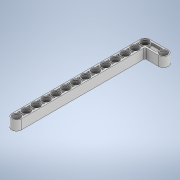
# Autodesk Inventor part: gear-rack
Saved by Autodesk Inventor 2021 (Build 250183000, 183)
## iProperties
Created: 2024-04-11
Part Number: gear-rack
Material: Generic
Document SubType Name: Modeling
Designer: 22hamfri
Density: 1 g/cm^3
Appearance: Default
Author: 22hamfri
Autodesk Inventor part; units mm, degrees
ref_plane "YZ Plane" through (0, 0, 0) normal (1, 0, 0) x (0, 1, 0)
ref_plane "XZ Plane" through (0, 0, 0) normal (0, 1, 0) x (-1, 0, 0)
ref_plane "XY Plane" through (0, 0, 0) normal (0, 0, 1) x (1, 0, 0)
sketch "Sketch1" plane through (0, 0, 0) normal (0, 1, 0) x (-1, 0, 0)
  circle A0 centre (0, 0) radius 2.575
  circle A1 centre (0, 0) radius 3.1
  circle A2 centre (0, 0) radius 3.8
  circle A3 centre (-14.94, 0) radius 2.575
  circle A4 centre (-14.94, 0) radius 3.1
  circle A5 centre (-14.94, 0) radius 3.8
  line L0 (0, -3.8) -> (-14.94, -3.8)
  line L1 (-4.8, 3.8) -> (-14.94, 3.8)
  line L2 (0, 0) -> (-14.94, 0)
  line L3 (0, 0) -> (0, 103.61)
  circle A6 centre (0, 7.97) radius 2.575
  circle A7 centre (0, 7.97) radius 3.1
  circle A8 centre (0, 7.97) radius 3.8
  circle A9 centre (0, 15.94) radius 2.575
  circle A10 centre (0, 15.94) radius 3.1
  circle A11 centre (0, 15.94) radius 3.8
  circle A12 centre (0, 23.91) radius 2.575
  circle A13 centre (0, 23.91) radius 3.1
  circle A14 centre (0, 23.91) radius 3.8
  circle A15 centre (0, 31.88) radius 2.575
  circle A16 centre (0, 31.88) radius 3.1
  circle A17 centre (0, 31.88) radius 3.8
  circle A18 centre (0, 39.85) radius 2.575
  circle A19 centre (0, 39.85) radius 3.1
  circle A20 centre (0, 39.85) radius 3.8
  circle A21 centre (0, 47.82) radius 2.575
  circle A22 centre (0, 47.82) radius 3.1
  circle A23 centre (0, 47.82) radius 3.8
  circle A24 centre (0, 55.79) radius 2.575
  circle A25 centre (0, 55.79) radius 3.1
  circle A26 centre (0, 55.79) radius 3.8
  circle A27 centre (0, 63.76) radius 2.575
  circle A28 centre (0, 63.76) radius 3.1
  circle A29 centre (0, 63.76) radius 3.8
  circle A30 centre (0, 71.73) radius 2.575
  circle A31 centre (0, 71.73) radius 3.1
  circle A32 centre (0, 71.73) radius 3.8
  circle A33 centre (0, 79.7) radius 2.575
  circle A34 centre (0, 79.7) radius 3.1
  circle A35 centre (0, 79.7) radius 3.8
  circle A36 centre (0, 87.67) radius 2.575
  circle A37 centre (0, 87.67) radius 3.1
  circle A38 centre (0, 87.67) radius 3.8
  circle A39 centre (0, 95.64) radius 2.575
  circle A40 centre (0, 95.64) radius 3.1
  circle A41 centre (0, 95.64) radius 3.8
  circle A42 centre (0, 103.61) radius 2.575
  circle A43 centre (0, 103.61) radius 3.1
  circle A44 centre (0, 103.61) radius 3.8
  line L4 (3.8, 103.61) -> (3.8, 0)
  line L5 (-3.8, 4.8) -> (-3.8, 103.61)
  line L6 (-3.0249, -2.3) -> (-11.9151, -2.3)
  line L7 (-3.0249, 2.3) -> (-11.9151, 2.3)
  line L8 (-2.3, 100.5851) -> (-2.3, 98.6649)
  line L9 (-2.3, 92.6151) -> (-2.3, 90.6949)
  line L10 (-2.3, 84.6451) -> (-2.3, 82.7249)
  line L11 (-2.3, 76.6751) -> (-2.3, 74.7549)
  line L12 (-2.3, 68.7051) -> (-2.3, 66.7849)
  line L13 (-2.3, 60.7351) -> (-2.3, 58.8149)
  line L14 (-2.3, 52.7651) -> (-2.3, 50.8449)
  line L15 (-2.3, 44.7951) -> (-2.3, 42.8749)
  line L16 (-2.3, 36.8251) -> (-2.3, 34.9049)
  line L17 (-2.3, 28.8551) -> (-2.3, 26.9349)
  line L18 (-2.3, 20.8851) -> (-2.3, 18.9649)
  line L19 (-2.3, 12.9151) -> (-2.3, 10.9949)
  line L20 (-2.3, 4.9451) -> (-2.3, 3.0249)
  line L21 (2.3, 100.5851) -> (2.3, 98.6649)
  line L22 (2.3, 92.6151) -> (2.3, 90.6949)
  line L23 (2.3, 84.6451) -> (2.3, 82.7249)
  line L24 (2.3, 76.6751) -> (2.3, 74.7549)
  line L25 (2.3, 68.7051) -> (2.3, 66.7849)
  line L26 (2.3, 60.7351) -> (2.3, 58.8149)
  line L27 (2.3, 52.7651) -> (2.3, 50.8449)
  line L28 (2.3, 44.7951) -> (2.3, 42.8749)
  line L29 (2.3, 36.8251) -> (2.3, 34.9049)
  line L30 (2.3, 28.8551) -> (2.3, 26.9349)
  line L31 (2.3, 20.8851) -> (2.3, 18.9649)
  line L32 (2.3, 12.9151) -> (2.3, 10.9949)
  line L33 (2.3, 4.9451) -> (2.3, 3.0249)
  arc A45 (-4.8, 3.8) -> (-3.8, 4.8) centre (-4.8, 4.8) ccw
  point P0 (0, 3.8)
  point P1 (0, 4.17)
  point P2 (0, 11.77)
  point P3 (0, 12.14)
  point P4 (0, 19.74)
  point P5 (0, 20.11)
  point P6 (0, 27.71)
  point P7 (0, 28.08)
  point P8 (0, 35.68)
  point P9 (0, 36.05)
  point P10 (0, 43.65)
  point P11 (0, 44.02)
  point P12 (0, 51.62)
  point P13 (0, 51.99)
  point P14 (0, 59.59)
  point P15 (0, 59.96)
  point P16 (0, 67.56)
  point P17 (0, 67.93)
  point P18 (0, 75.53)
  point P19 (0, 75.9)
  point P20 (0, 83.5)
  point P21 (0, 83.87)
  point P22 (0, 91.47)
  point P23 (0, 91.84)
  point P24 (0, 99.44)
  point P25 (0, 99.81)
  point P26 (0, 107.41)
  point P27 (-3.8, 0)
  dimension "d0" = 0.7
  dimension "d1" = 6.2
  dimension "d2" = 5.15
  dimension "d3" = 5.15
  dimension "d4" = 6.2
  dimension "d5" = 0.7
  dimension "d6" = 14.94
  dimension "d9" = 7.97
  dimension "d14" = 1.5
  dimension "d15" = 1.5
  dimension "d16" = 1.5
  dimension "d17" = 1
  constraints: 68 end point, 59 point on circle, 51 point on line, 45 centre point, 26 symmetric about line, 6 tangent, 4 vertical, 3 horizontal, 2 coincident, 2 parallel, 1 line through centre, 86 other
  measures "d1" diameter of A1
  measures "d2" diameter of A0
  measures "d3" diameter of A3
  measures "d4" diameter of A4
  measures "d5" radial gap between concentric circles of A4 A5
  measures "d6" distance of L2.start L2.end
  measures "d9" distance of L2.start A6.centre
  measures "d14" distance between parallel lines of L0 L6
  measures "d15" distance between parallel lines of L1 L7
  measures "d16" distance between parallel lines of L19 L5
  measures "d17" radius of A45
extrude "Extrusion1" add sketch "Sketch1" against normal mid plane 7.76 contours L3 A2 L2 A1 | A1 L2 A2 L3 | L33 A8 L4 A2 | A2 L7 A5 L1 A45 L5 A8 L20 | A8 L3 A7 | L3 A7 A8 | A2 L0 A5 L6 | A5 | A8 L32 A11 L4 | L5 A11 L19 A8 | A11 L3 A10 | A11 L31 A14 L4 | L5 A14 L18 A11 | A11 L3 A10 | A14 L3 A13 | A14 L30 A17 L4 | L5 A17 L17 A14 | A14 L3 A13 | A17 L3 A16 | A17 L29 A20 L4 | L5 A20 L16 A17 | A17 L3 A16 | A20 L3 A19 | A20 L28 A23 L4 | L5 A23 L15 A20 | A20 L3 A19 | A23 L3 A22 | A23 L27 A26 L4 | L5 A26 L14 A23 | A23 L3 A22 | A26 L3 A25 | A26 L26 A29 L4 | L5 A29 L13 A26 | A26 L3 A25 | A29 L3 A28 | A29 L25 A32 L4 | L5 A32 L12 A29 | A29 L3 A28 | A32 L3 A31 | A32 L24 A35 L4 | L5 A35 L11 A32 | A32 L3 A31 | A35 L3 A34 | A35 L23 A38 L4 | L5 A38 L10 A35 | A35 L3 A34 | A38 L3 A37 | A38 L22 A41 L4 | L5 A41 L9 A38 | A38 L3 A37 | A41 L3 A40 | A41 L21 A44 L4 | L5 A44 L8 A41 | A41 L3 A40 | A44
extrude "Extrusion2" add sketch "Sketch1" against normal mid plane 6.16 contours A0 L3 A1 L2 | A0 L2 A1 L3 | A4 | A7 L3 A6 | L3 A6 A7 | A10 L3 A9 | L3 A9 A10 | A13 L3 A12 | L3 A12 A13 | A16 L3 A15 | L3 A15 A16 | A19 L3 A18 | L3 A18 A19 | A22 L3 A21 | L3 A21 A22 | A25 L3 A24 | L3 A24 A25 | A28 L3 A27 | L3 A27 A28 | A31 L3 A30 | L3 A30 A31 | A34 L3 A33 | L3 A33 A34 | A43 | A37 L3 A36 | L3 A36 A37 | A40 L3 A39 | L3 A39 A40
extrude "Extrusion3" add sketch "Sketch1" against normal mid plane 4 contours L3 A8 L33 A2 | A2 L20 A8 L3 | L2 A5 L7 A2 | A2 L6 A5 L2 | A8 L3 A11 L32 | L19 A11 L3 A8 | A11 L3 A14 L31 | L18 A14 L3 A11 | A14 L3 A17 L30 | L17 A17 L3 A14 | A17 L3 A20 L29 | L16 A20 L3 A17 | A20 L3 A23 L28 | L15 A23 L3 A20 | A23 L3 A26 L27 | L14 A26 L3 A23 | A26 L3 A29 L26 | L13 A29 L3 A26 | A29 L3 A32 L25 | L12 A32 L3 A29 | A32 L3 A35 L24 | L11 A35 L3 A32 | A35 L3 A38 L23 | L10 A38 L3 A35 | A38 L3 A41 L22 | L9 A41 L3 A38 | A41 L3 A44 L21 | L8 A44 L3 A41
body "Solid1"
